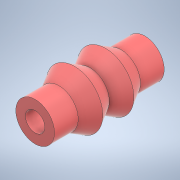
# Autodesk Inventor part: Flex
Saved by Autodesk Inventor 2022 (Build 260153000, 153)
## iProperties
Created: 2021-11-09
Part Number: Flex
Material: Generic
Document SubType Name: Modeling
Designer: Juan
Density: 1 g/cm^3
Appearance: Default
Author: Juan
Autodesk Inventor part; units mm, degrees
ref_plane "YZ Plane" through (0, 0, 0) normal (1, 0, 0) x (0, 1, 0)
ref_plane "XZ Plane" through (0, 0, 0) normal (0, 1, 0) x (-1, 0, 0)
ref_plane "XY Plane" through (0, 0, 0) normal (0, 0, 1) x (1, 0, 0)
sketch "Sketch1" plane through (0, 0, 0) normal (1, 0, 0) x (0, 1, 0)
  line L0 (0, 0) -> (0, 8.5)
  line L1 (0, 8.5) -> (3, 8.5)
  line L2 (3, 0) -> (4.3916, 2.4103)
  line L3 (3, 0) -> (5.7832, 0) construction
  line L4 (4.3916, 2.4103) -> (3, 4.8207)
  line L5 (3, 0) -> (0, 0)
  line L6 (3, 8.5) -> (3, 7.5231)
  line L7 (3, 7.5231) -> (3, 4.8207)
  dimension "d0" = 8.5
  dimension "d1" = 3
  dimension "d3" = 60
  dimension "d4" = 120
  constraints: 16 end point, 2 equal length, 2 horizontal, 2 perpendicular, 1 point on line, 1 vertical
  measures "d0" distance of L0.start L0.end
  measures "d1" distance of L0.end L1.end
  measures "d3" angle of L3 L2
  measures "d4" angle of L4 L2
revolve "Revolution1" add sketch "Sketch1" angle 360 about axis through (0, 0, 0) along (0, 0, 1)
mirror "Mirror1" about plane through (0, 0, 0) normal (0, 0, -1)
shell "Shell1" thickness 1.5 removed faces 2 at (-1.0949, -0.5351, 8.5) at (-1.0949, -0.5351, -8.5)
body "Solid1"
